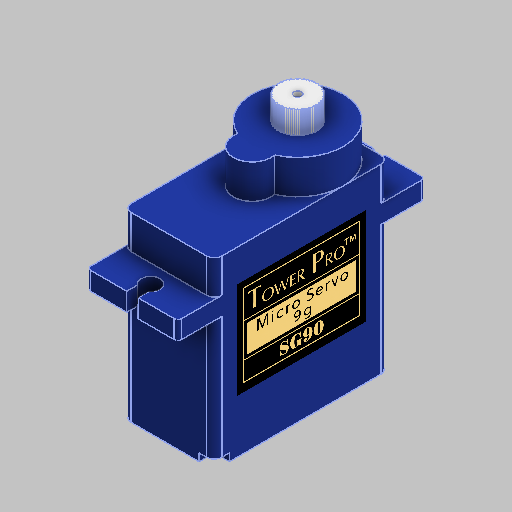
# Autodesk Inventor part: SERVO_SG90
Saved by Autodesk Inventor 2026 (Build 300175000, 175)
## iProperties
Created: 2026-06-09
Part Number: SERVO_SG90
Material: Plástico PC/ABS
Document SubType Name: Modeling
Designer: mathe
Density: 1.1 g/cm^3
Appearance: Padrão(1)
Author: mathe
Autodesk Inventor part; units mm, degrees
ref_plane "YZ Plane" through (0, 0, 0) normal (1, 0, 0) x (0, 1, 0)
ref_plane "XZ Plane" through (0, 0, 0) normal (0, 1, 0) x (-1, 0, 0)
ref_plane "XY Plane" through (0, 0, 0) normal (0, 0, 1) x (1, 0, 0)
sketch "Esboço1" plane through (0, 0, 0) normal (0, 1, 0) x (-1, 0, 0)
  line L0 (-6, -11.5) -> (6, -11.5)
  line L1 (6, -11.5) -> (6, 11.5)
  line L2 (6, 11.5) -> (-6, 11.5)
  line L3 (-6, 11.5) -> (-6, -11.5)
  line L4 (-6, -11.5) -> (6, 11.5) construction
  line L5 (6, -11.5) -> (-6, 11.5) construction
  point P0 (0, 0)
  dimension "d0" = 12
  dimension "d1" = 23
  constraints: 12 end point, 2 midpoint, 2 parallel, 1 horizontal, 1 perpendicular
  measures "d0" distance of L2.end L1.end
  measures "d1" distance of L1.end L0.end
extrude "Extrusão1" add sketch "Esboço1" along normal blind 24
sketch "Esboço2" plane through (-6, 0, 11.5) normal (0, 0, 1) x (1, 0, 0)
  line L0 (0, 0) -> (0, 24) projected
  line L1 (12, 0) -> (12, 24) projected
  line L2 (0, 17.1) -> (12, 17.1)
  line L3 (12, 17.1) -> (12, 19.5)
  line L4 (12, 19.5) -> (0, 19.5)
  line L5 (0, 19.5) -> (0, 17.1)
  line L6 (0, 24) -> (12, 24) projected
  point P0 (6, 0)
  point P1 (0, 19.5)
  dimension "d4" = 2.4
  dimension "d5" = 4.5
  constraints: 8 end point, 2 parallel, 2 point on line, 1 horizontal, 1 perpendicular
  measures "d4" distance of L3.end L2.end
  measures "d5" distance between parallel lines of L4 L6
extrude "Extrusão2" add sketch "Esboço2" along normal blind 4.8 contours L0 L4 L1 L2
sketch "Esboço3" plane through (-6, 19.5, 11.5) normal (0, 1, 0) x (1, 0, 0)
  line L0 (0, -4.8) -> (12, -4.8) projected
  line L1 (6, -4.8) -> (6, 0)
  line L2 (12, 0) -> (0, 0) projected
  arc A0 (6.75, -3.4) -> (5.25, -3.4) centre (6, -2.4) ccw
  line L3 (6.75, -4.8) -> (5.25, -4.8)
  line L4 (5.25, -4.8) -> (5.25, -3.4)
  line L5 (6.75, -3.4) -> (6.75, -4.8)
  line L6 (12, -4.8) -> (0, -4.8) projected
  point P0 (6, 11.5)
  dimension "d8" = 2.5
  constraints: 8 end point, 5 midpoint, 2 point on circle, 1 centre point, 1 horizontal, 1 parallel, 1 perpendicular
  measures "d8" diameter of A0
extrude "Extrusão3" cut sketch "Esboço3" against normal through all
fillet "Arredondamento1" radius 0.5 2 edges at (6, 18.3, 16.3) (-6, 18.3, 16.3)
mirror "Espelhar1" about plane through (0, 0, 0) normal (0, 0, 1) of "Extrusão2", "Extrusão3", "Arredondamento1"
sketch "Esboço6" plane through (0, 24, 0) normal (0, 1, 0) x (1, 0, 0)
  circle A0 centre (0, 5.5) radius 6
  circle A1 centre (0, -0.5) radius 2.5
  line L0 (6, 11.5) -> (-6, 11.5) projected
  point P0 (0, 0)
  point P1 (0, -3)
  point P2 (0, 11.5)
  point P3 (-2.4451, 0.0208)
  point P4 (2.4451, 0.0208)
  dimension "d27" = 12
  dimension "d28" = 5
  dimension "d29" = 14.5
  constraints: 2 vertical alignment, 1 midpoint, 6 other
  measures "d29" distance of point (0, 11.5) point (0, -3)
extrude "Extrusão6" add sketch "Esboço6" along normal blind 4.5
sketch "Esboço7" plane through (0, 28.5, 0) normal (0, 1, 0) x (1, 0, 0)
  arc A0 (0, 11.5) -> (-6, 5.5) centre (0, 5.5) ccw projected
  circle A1 centre (0, 5.5) radius 2.5
  point P0 (0, 0)
  dimension "d32" = 5
  constraints: 1 centre point, 1 coincident
  measures "d32" diameter of A1
extrude "Extrusão7" add sketch "Esboço7" along normal blind 3 separate body
sketch "Esboço9" plane through (0, 31.5, -5.5) normal (0, 1, 0) x (1, 0, 0)
  circle A0 centre (0, 0) radius 2.5 projected
  circle A1 centre (0, -2.5) radius 0.1
  point P0 (0, -5.5)
  point P1 (0.1, -2.498)
  point P2 (-0.1, -2.498)
  dimension "d38" = 0.2
  constraints: 1 centre point, 2 other
  measures "d38" diameter of A1
extrude "Extrusão9" cut sketch "Esboço9" against normal up to surface (3 mm away) contours A0 A1 picked at (-0.0071, -2.4673) bodies 2
pattern_circular "Padrão circular1" count 40 over 360 about axis through (0, 28.5, -5.5) along (0, 1, 0) of "Extrusão9" bodies 2
sketch "Esboço10" plane through (0, 31.5, 0) normal (0, 1, 0) x (1, 0, 0)
  arc A0 (2.4829, 5.208) -> (2.498, 5.4) centre (0, 5.5) ccw projected
  circle A1 centre (0, 5.5) radius 0.5
  point P0 (0, 0)
  dimension "d44" = 1
  constraints: 1 centre point, 1 coincident
  measures "d44" diameter of A1
extrude "Extrusão10" cut sketch "Esboço10" against normal up to surface (3 mm away) bodies 2
sketch "Esboço11" plane through (0, 0, 0) normal (0, -1, 0) x (1, 0, 0)
  line L0 (-6, -11.5) -> (6, -11.5) projected
  line L1 (-6, -11.5) -> (-4, -11.5)
  line L2 (-4, -11.5) -> (-4, -10.5)
  line L3 (-5, -9.5) -> (-6, -9.5)
  line L4 (-6, -9.5) -> (-6, -11.5)
  arc A0 (-4, -10.5) -> (-5, -9.5) centre (-5, -10.5) ccw
  line L5 (-6, 11.5) -> (6, 11.5) projected
  line L6 (6, 11.5) -> (4, 11.5)
  line L7 (4, 11.5) -> (4, 10.5)
  line L8 (5, 9.5) -> (6, 9.5)
  line L9 (6, 9.5) -> (6, 11.5)
  arc A1 (4, 10.5) -> (5, 9.5) centre (5, 10.5) ccw
  point P0 (0, 0)
  point P1 (-4, -9.5)
  point P2 (4, 9.5)
  dimension "d47" = 2
  dimension "d48" = 2
  dimension "d49" = 1
  dimension "d50" = 2
  dimension "d51" = 2
  dimension "d52" = 1
  constraints: 16 end point, 4 parallel, 4 point on circle, 4 point on line, 4 tangent, 2 centre point, 2 horizontal, 2 perpendicular
  measures "d47" distance of L3.end point (-4, -9.5)
  measures "d48" distance of point (-4, -9.5) L1.end
  measures "d49" radius of A0
  measures "d50" distance of L8.end point (4, 9.5)
  measures "d51" distance of point (4, 9.5) L6.end
  measures "d52" radius of A1
extrude "Extrusão11" cut sketch "Esboço11" against normal blind 1 bodies 1
fillet "Arredondamento3" radius 1 8 edges at (-6, 8.55, 11.5) (6, 9.05, 11.5) (-6, 21.75, 11.5) (6, 21.75, 11.5) (-6, 21.75, -11.5) (-6, 9.05, -11.5) (6, 21.75, -11.5) (6, 8.55, -11.5)
sketch "Esboço12" plane through (0, 0, 0) normal (0, -1, 0) x (1, 0, 0)
  line L0 (5, -11.5) -> (-4, -11.5) projected
  line L1 (1.8, -11.5) -> (-1.8, -11.5)
  line L2 (-1.8, -11.5) -> (-1.8, -10)
  line L3 (-1.8, -10) -> (1.8, -10)
  line L4 (1.8, -10) -> (1.8, -11.5)
  arc A0 (0.75, -14.9) -> (-0.75, -14.9) centre (0, -13.9) ccw projected
  point P0 (0, 0)
  point P1 (0, -11.5)
  point P2 (0, -12.65)
  dimension "d56" = 3.6
  dimension "d57" = 1.5
  constraints: 8 end point, 2 parallel, 1 horizontal, 1 midpoint, 1 perpendicular, 1 point on circle, 1 point on line, 1 vertical alignment
  measures "d56" distance of L2.end L3.end
  measures "d57" distance of L1.end L2.end
extrude "Extrusão12" cut sketch "Esboço12" against normal blind 5 bodies 1
sketch "Esboço13" plane through (1.8, 0, -10) normal (0, 0, -1) x (-1, 0, 0)
  line L0 (0, 5) -> (3.6, 5) projected
  line L1 (0, 5) -> (0, 4.4)
  line L2 (0, 0) -> (0, 5) projected
  line L3 (0, 4.4) -> (0.6, 4.4)
  circle A0 centre (0.6, 4.4) radius 0.6
  point P0 (1.8, 0)
  dimension "d60" = 0.6
  dimension "d61" = 0.6
  dimension "d62" = 1.2
  constraints: 4 end point, 1 centre point, 1 coincident, 1 horizontal, 1 point on line
  measures "d60" distance of L0.start L1.end
  measures "d61" distance of L1.end L3.end
  measures "d62" diameter of A0
extrude "Extrusão13" add sketch "Esboço13" along normal blind 5 separate body contours A0
sketch "Esboço14" plane through (1.8, 0, -10) normal (0, 0, -1) x (-1, 0, 0)
  circle A0 centre (1.8, 4.4) radius 0.6
  circle A1 centre (0.6, 4.4) radius 0.6 projected
  point P0 (1.8, 0)
  dimension "d65" = 1.2
  dimension "d66" = 1.2
  constraints: 1 centre point
  measures "d65" diameter of A0
  measures "d66" distance of A1.centre A0.centre
extrude "Extrusão14" add sketch "Esboço14" along normal blind 5 separate body contours A0
sketch "Esboço15" plane through (1.8, 0, -10) normal (0, 0, -1) x (-1, 0, 0)
  circle A0 centre (1.8, 4.4) radius 0.6 projected
  line L0 (1.8, 4.4) -> (3, 4.4)
  circle A1 centre (3, 4.4) radius 0.6
  point P0 (1.8, 0)
  dimension "d69" = 1.2
  dimension "d70" = 1.2
  constraints: 2 end point, 1 centre point, 1 coincident, 1 horizontal
  measures "d69" distance of L0.start L0.end
  measures "d70" diameter of A1
extrude "Extrusão15" add sketch "Esboço15" along normal blind 5 separate body contours A1
sketch "Esboço16" plane through (6, 17.1, 15.8) normal (1, 0, 0) x (0, 0, -1)
  line L0 (7.3, 2.65) -> (24.3, 2.65) construction
  line L1 (24.3, 2.65) -> (24.3, -10.1) construction
  line L2 (24.3, -10.1) -> (7.3, -10.1) construction
  line L3 (7.3, -10.1) -> (7.3, 2.65) construction
  line L4 (6.3, -17.1) -> (26.3, -17.1) projected
  point P0 (15.8, -17.1)
  point P1 (15.8, -10.1)
  dimension "d74" = 17
  dimension "d80" = 7
  constraints: 1 midpoint, 1 vertical alignment, 2 other
  measures "d74" distance of L0.start L0.end
  measures "d80" distance between parallel lines of L4 L2
decal "Decalque1"
sketch "Esboço17" plane through (-6, 17.1, 15.8) normal (-1, 0, 0) x (0, 0, 1)
  line L0 (-23.8, 2.65) -> (-6.8, 2.65) construction
  line L1 (-6.8, 2.65) -> (-6.8, -10.1) construction
  line L2 (-6.8, -10.1) -> (-23.8, -10.1) construction
  line L3 (-23.8, -10.1) -> (-23.8, 2.65) construction
  line L4 (-25.3, -17.1) -> (-5.3, -17.1) projected
  point P0 (-15.8, -17.1)
  point P1 (-15.3, -10.1)
  point P2 (-15.3, -17.1)
  dimension "d82" = 17
  dimension "d88" = 7
  constraints: 2 midpoint, 1 vertical alignment, 2 other
  measures "d82" distance of L0.start L0.end
  measures "d88" distance between parallel lines of L4 L2
decal "Decalque2"
